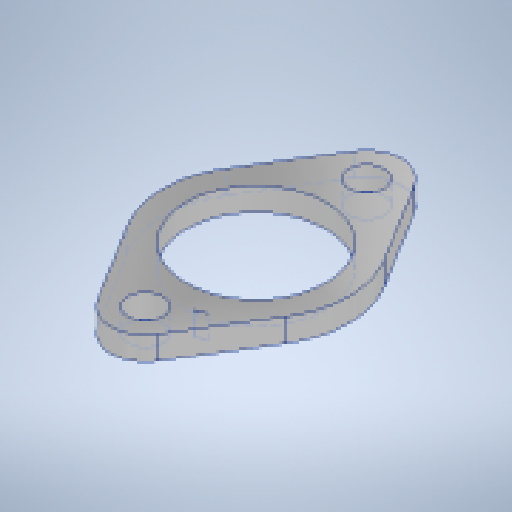
# Autodesk Inventor part: tension2
Saved by Autodesk Inventor 2025 (Build 290162000, 162)
## iProperties
Created: 2025-03-05
Part Number: tension2
Material: アルミニウム 6061
Document SubType Name: Modeling
Designer: Zhopa
Density: 2.7 g/cm^3
Appearance: アルミニウム - フラット
Mass: 0.754388 g
Surface Area: 5.20889 cm^2
Volume: 0.279403 cm^3
Author: Zhopa
Autodesk Inventor part; units mm, degrees
ref_plane "YZ Plane" through (0, 0, 0) normal (1, 0, 0) x (0, 1, 0)
ref_plane "XZ Plane" through (0, 0, 0) normal (0, 1, 0) x (-1, 0, 0)
ref_plane "XY Plane" through (0, 0, 0) normal (0, 0, 1) x (1, 0, 0)
sketch "Sketch1" plane through (0, 0, 0) normal (0, 1, 0) x (-1, 0, 0)
  circle A0 centre (0, 0) radius 6
  circle A1 centre (0, -9.5) radius 1.5
  circle A2 centre (0, 9.5) radius 1.5
  circle A3 centre (0, 9.5) radius 3
  circle A4 centre (0, -9.5) radius 3
  circle A5 centre (0, 0) radius 8
  line L0 (2.5509, 11.0789) -> (6.8023, 4.2105)
  line L1 (0, 0) -> (6, 0)
  line L2 (2.5509, -11.0789) -> (6.8023, -4.2105)
  line L3 (4.132, 10.5914) -> (-3.2494, 7.3104)
  line L4 (-8.0078, 0) -> (-7.9923, 0.3519)
  line L5 (-2.5509, 11.0789) -> (-6.8023, 4.2105)
  line L6 (-6.8023, -4.2105) -> (-2.5509, -11.0789)
  point P0 (2.9464, 10.0644)
  point P1 (-3.2494, 7.3104)
  point P2 (-7.9923, 0.3519)
  point P3 (-2.6722, -12.3636)
  point P4 (2.5509, -11.0789)
  point P5 (6.8023, -4.2105)
  point P6 (-2.3575, 7.6447)
  point P7 (2.3575, 7.6447)
  point P8 (3.1287, 10.1454)
  point P9 (-2.3932, 7.6909)
  point P10 (-2.3575, -7.6447)
  point P11 (2.3575, -7.6447)
  point P12 (1.4979, 9.4205)
  point P13 (0, 8)
  point P14 (0, -8)
  point P15 (-0.9446, 8.3348)
  dimension "d2" = 12
  dimension "d6" = 6
  dimension "d0" = 9.5
  dimension "d1" = 9.5
  dimension "d3" = 3
  dimension "d4" = 3
  dimension "d5" = 6
  dimension "d7" = 16
  constraints: 14 end point, 7 coincident, 5 point on circle, 4 centre point, 3 tangent, 2 symmetric about line, 1 horizontal, 1 horizontal alignment, 1 point on line, 6 other
  measures "d0" distance of point (0, -9.5) point (0, 0)
  measures "d1" distance of point (0, 9.5) point (0, 0)
  measures "d3" diameter of A1
  measures "d4" diameter of A2
  measures "d5" diameter of A3
  measures "d7" diameter of A5
extrude "Extrusion1" add sketch "Sketch1" along normal blind 2 contours A5 A4 | A5 A4 | A5 A3 A4 | A4 L6 A5 | A5 L2 A4 | L5 A3 L3 A5 | A5 A3 L3 L0 | A3 L3 A2 | A5 A2 L3 A3 | A3 A5 | L3 A3 L0 | A3 L3 A2 A5
body "Solid1"
